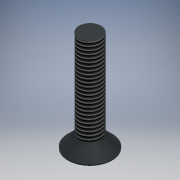
# Autodesk Inventor part: M5皿ネジ 20
Saved by Autodesk Inventor 2017.3 (Build 213256000, 256)
## iProperties
Part Number: M5皿ネジ 20
Material: 鉄 灰色
Document SubType Name: Modeling
Designer: 原知也
Density: 7.15 g/cm^3
Appearance: 鉄 灰色
Author: 原知也
Autodesk Inventor part; units mm, degrees
ref_plane "YZ Plane" through (0, 0, 0) normal (1, 0, 0) x (0, 1, 0)
ref_plane "XZ Plane" through (0, 0, 0) normal (0, 1, 0) x (-1, 0, 0)
ref_plane "XY Plane" through (0, 0, 0) normal (0, 0, 1) x (1, 0, 0)
sketch "スケッチ1" plane through (0, 0, 0) normal (0, 0, 1) x (1, 0, 0)
  circle A0 centre (0, 0) radius 2.5
  dimension "d0" = 5
  constraints: 1 centre point, 1 coincident
  measures "d0" diameter of A0
extrude "押し出し1" add sketch "スケッチ1" along normal blind 20
sketch "スケッチ2" plane through (0, 0, 0) normal (0, 0, -1) x (-1, 0, 0)
  circle A0 centre (0, 0) radius 5
  dimension "d3" = 10
  constraints: 1 centre point, 1 coincident
  measures "d3" diameter of A0
extrude "押し出し2" add sketch "スケッチ2" along normal blind 2.8
chamfer "面取り1" distance 2.5 angle 45 1 edges at (5, 0, 0)
sketch "スケッチ3" plane through (0, 0, -2.8) normal (0, 0, -1) x (-1, 0, 0)
  line L0 (0, 1.7321) -> (1.5, 0.866)
  line L1 (1.5, 0.866) -> (1.5, -0.866)
  line L2 (1.5, -0.866) -> (0, -1.7321)
  line L3 (0, -1.7321) -> (-1.5, -0.866)
  line L4 (-1.5, -0.866) -> (-1.5, 0.866)
  line L5 (-1.5, 0.866) -> (0, 1.7321)
  point P0 (0, 0)
  point P1 (0, 0)
  dimension "d12" = 3
  constraints: 12 end point, 1 coincident, 13 other
  measures "d12" distance between parallel lines of L3 L0
extrude "押し出し3" cut sketch "スケッチ3" against normal blind 2.5
thread "ねじ1" size "M5x0.8" class "6g" standard "ANSI Metric M Profile" full length
